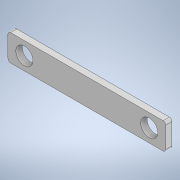
# Autodesk Inventor part: rodFixer
Saved by Autodesk Inventor 2021 (Build 250183000, 183)
## iProperties
Created: 2022-09-09
Part Number: rodFixer
Material: Generic
Document SubType Name: Modeling
Designer: szucs
Density: 1 g/cm^3
Appearance: Default
Author: szucs
Autodesk Inventor part; units mm, degrees
ref_plane "YZ Plane" through (0, 0, 0) normal (1, 0, 0) x (0, 1, 0)
ref_plane "XZ Plane" through (0, 0, 0) normal (0, 1, 0) x (-1, 0, 0)
ref_plane "XY Plane" through (0, 0, 0) normal (0, 0, 1) x (1, 0, 0)
sketch "Sketch1" plane through (0, 0, 0) normal (0, 0, 1) x (1, 0, 0)
  line L0 (0, 14) -> (0, -14) projected
  line L1 (-84, 0) -> (84, 0) projected
  line L2 (-60, 10) -> (60, 10)
  line L3 (60, 10) -> (60, -10)
  line L4 (60, -10) -> (-60, -10)
  line L5 (-60, -10) -> (-60, 10)
  point P0 (0, 0)
  dimension "d0" = 120
  dimension "d1" = 20
  constraints: 8 end point, 2 parallel, 1 horizontal, 1 perpendicular, 2 other
  measures "d0" distance of L3.end L4.end
  measures "d1" distance of L4.end L2.start
extrude "Extrusion1" add sketch "Sketch1" along normal blind 4.8
sketch "Sketch2" plane through (0, 0, 4.8) normal (0, 0, 1) x (1, 0, 0)
  line L0 (-60, -10) -> (60, -10) projected
  line L1 (60, -10) -> (60, 10) projected
  line L2 (60, 10) -> (-60, 10) projected
  line L3 (-60, 10) -> (-60, -10) projected
  circle A0 centre (-47.5, 0) radius 6.5
  circle A1 centre (47.5, 0) radius 6.5
  line L4 (0, 14) -> (0, -14) projected
  point P0 (0, 0)
  dimension "d4" = 13
  dimension "d5" = 13
  dimension "d6" = 95
  constraints: 2 centre point, 1 symmetric about line
  measures "d4" diameter of A0
  measures "d5" diameter of A1
  measures "d6" distance of A1.centre A0.centre
extrude "Extrusion2" cut sketch "Sketch2" against normal through all contours A0 | A1
fillet "Fillet1" radius 2 4 edges at (-60, 10, 2.4) (-60, -10, 2.4) (60, 10, 2.4) (60, -10, 2.4)
body "Solid1"
